Autodesk Fusion 360 part; units mm, degrees
note: some values were not read from the file. Set by a fixed rule: which sketch regions a step uses.
(part 2 of 2)
sketch "Sketch29" plane through (0, 0, 0) normal (0, -1, 0) x (1, 0, 0)
  circle A0 centre (-29.9934, -95.0047) radius 5
  arc A1 (-9.95, -103.9) -> (-9.7099, -104.5501) centre (-8.95, -103.9) ccw
  line L0 (-9.95, -103.9) -> (-9.95, -99.8)
  arc A2 (-8.95, -98.8) -> (-9.95, -99.8) centre (-8.95, -99.8) ccw
  line L1 (-8.95, -98.8) -> (8.95, -98.8)
  arc A3 (9.95, -99.8) -> (8.95, -98.8) centre (8.95, -99.8) ccw
  line L2 (9.95, -99.8) -> (9.95, -103.9)
  arc A4 (9.7099, -104.5501) -> (9.95, -103.9) centre (8.95, -103.9) ccw
  arc A5 (9.7099, -104.5501) -> (98.5902, -36.1245) centre (0, 0) ccw
  arc A6 (98.5902, -36.1245) -> (96.7123, -33.4364) centre (96.7123, -35.4364) ccw
  line L3 (96.7123, -33.4364) -> (85, -33.4364)
  line L4 (85, -33.4364) -> (85, -31.5073)
  line L5 (85, -31.5073) -> (75, -31.5073)
  line L6 (75, -31.5073) -> (75, -23.5073)
  line L7 (75, -23.5073) -> (74.9628, -23.5073)
  line L8 (74.9628, -23.5073) -> (74.9628, -27.0073)
  line L9 (74.9628, -27.0073) -> (34.9628, -27.0073)
  line L10 (34.9628, -27.0073) -> (34.9628, -21.5073)
  line L11 (34.9628, -21.5073) -> (31.9628, -21.5073)
  line L12 (31.9628, -21.5073) -> (31.9628, 21.4927)
  line L13 (31.9628, 21.4927) -> (34.9628, 21.4927)
  line L14 (34.9628, 21.4927) -> (34.9628, 21.5)
  line L15 (34.9628, 21.5) -> (-35.0372, 21.5)
  line L16 (-35.0372, 21.5) -> (-35.0372, 21.4927)
  line L17 (-35.0372, 21.4927) -> (-32.0372, 21.4927)
  line L18 (-32.0372, 21.4927) -> (-32.0372, -21.5073)
  line L19 (-32.0372, -21.5073) -> (-35.0372, -21.5073)
  line L20 (-35.0372, -21.5073) -> (-35.0372, -23.5073)
  line L21 (-35.0372, -23.5073) -> (-34.9628, -23.5073)
  line L22 (-34.9628, -23.5073) -> (-34.9628, -27.0073)
  line L23 (-34.9628, -27.0073) -> (-74.9628, -27.0073)
  line L24 (-74.9628, -27.0073) -> (-74.9628, -23.5073)
  line L25 (-74.9628, -23.5073) -> (-75, -23.5073)
  line L26 (-75, -23.5073) -> (-75, -31.5073)
  line L27 (-75, -31.5073) -> (-85, -31.5073)
  line L28 (-85, -31.5073) -> (-85, -33.4364)
  line L29 (-85, -33.4364) -> (-96.7123, -33.4364)
  arc A7 (-96.7123, -33.4364) -> (-98.5902, -36.1245) centre (-96.7123, -35.4364) ccw
  arc A8 (-98.5902, -36.1245) -> (-9.7099, -104.5501) centre (0, 0) ccw
  circle A9 centre (-14, -99) radius 2.1
  circle A10 centre (14, -99) radius 2.1
  line L30 (5, -90) -> (-5, -90)
  line L31 (-5, -90) -> (-5, -85)
  line L32 (-5, -85) -> (5, -85)
  line L33 (5, -85) -> (5, -90)
  circle A11 centre (-75, -37.0037) radius 4
  circle A12 centre (25, 11.9963) radius 4
  circle A13 centre (75, -37.0037) radius 4
  circle A14 centre (-25, 11.9963) radius 4
  circle A15 centre (13.6, -57.25) radius 1.35
  circle A16 centre (13.6, -29.45) radius 1.35
  circle A17 centre (38.8, -57.25) radius 1.35
  circle A18 centre (38.8, -29.45) radius 1.35
  line L34 (17.95, -68.0037) -> (17.95, -54.0037)
  arc A19 (17.95, -54) -> (17.95, -54.0037) centre (18.95, -54.0037) ccw
  line L35 (17.95, -54) -> (15, -54)
  arc A20 (14, -53) -> (15, -54) centre (15, -53) ccw
  line L36 (14, -53) -> (14, -41)
  arc A21 (15, -40) -> (14, -41) centre (15, -41) ccw
  line L37 (15, -40) -> (39, -40)
  arc A22 (40, -41) -> (39, -40) centre (39, -41) ccw
  line L38 (40, -41) -> (40, -53)
  arc A23 (39, -54) -> (40, -53) centre (39, -53) ccw
  line L39 (39, -54) -> (33.95, -54)
  arc A24 (33.95, -54.0037) -> (33.95, -54) centre (32.95, -54.0037) ccw
  line L40 (33.95, -54.0037) -> (33.95, -77.0037)
  arc A25 (32.95, -78.0037) -> (33.95, -77.0037) centre (32.95, -77.0037) ccw
  line L41 (32.95, -78.0037) -> (30, -78.0037)
  line L42 (30, -78.0037) -> (30, -86)
  arc A26 (29, -87) -> (30, -86) centre (29, -86) ccw
  line L43 (29, -87) -> (23, -87)
  arc A27 (22, -86) -> (23, -87) centre (23, -86) ccw
  line L44 (22, -86) -> (22, -83.0037)
  line L45 (22, -83.0037) -> (-18, -83.0037)
  arc A28 (-20, -81.0037) -> (-18, -83.0037) centre (-18, -81.0037) ccw
  line L46 (-20, -81.0037) -> (-20, -70.0037)
  arc A29 (-18, -68.0037) -> (-20, -70.0037) centre (-18, -70.0037) ccw
  line L47 (-18, -68.0037) -> (17.95, -68.0037)
  circle A30 centre (29.9934, -95.0047) radius 5
  line L48 (-35.6327, 21.4927) -> (-29.1327, 21.4927)
  line L49 (-29.1327, 21.4927) -> (-29.1327, -21.5073)
  line L50 (-29.1327, -21.5073) -> (-35.6327, -21.5073)
  line L51 (-35.6327, -21.5073) -> (-35.6327, 21.4927)
  line L52 (-35.0372, 21.4927) -> (-39.9159, 21.4927)
  line L53 (35.6068, 21.4927) -> (29.1068, 21.4927)
  line L54 (29.1068, 21.4927) -> (29.1068, -21.5073)
  line L55 (29.1068, -21.5073) -> (35.6068, -21.5073)
  line L56 (35.6068, -21.5073) -> (35.6068, 21.4927)
  line L57 (39.9159, 21.4927) -> (34.9628, 21.4927)
  dimension "d380" = 6.5
  dimension "d381" = 43
  dimension "d382" = 6.5
  dimension "d383" = 43
  constraint horizontal L48
  constraint vertical L49
  constraint horizontal L50
  constraint vertical L51
  constraint coincident L48.start L52
  constraint horizontal L53
  constraint vertical L54
  constraint horizontal L55
  constraint vertical L56
  constraint coincident L53.start L57
  measures "d380" distance of L48.start L48.end
  measures "d381" distance of L48.start L50.end
  measures "d382" distance of L53.start L53.end
  measures "d383" distance of L53.start L55.end
extrude "Extrude42" cut sketch "Sketch29" against normal blind 3 contours L17 L18 L19 L48 L50 L51 L52 | L18 L48 L49 L50 | L11 L12 L13 L53 L55 L56 L57 | L12 L53 L54 L55
equation "d285 = ( 43 / 2 ) * 1 mm"
